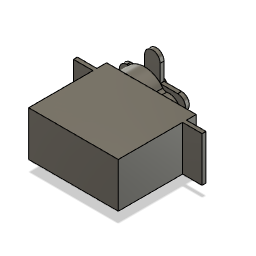
Pan_Tilt_Assembly (Autodesk Fusion 360 archive; units mm, degrees)
design "Servo9gr"
Autodesk Fusion 360 part; units mm, degrees
sketch "Skizze1" plane through (0, 0, 0) normal (0, 0, 1) x (1, 0, 0)
  line L0 (11.5, 5.75) -> (-11.5, 5.75)
  line L1 (-11.5, 5.75) -> (-11.5, -5.75)
  line L2 (-11.5, -5.75) -> (11.5, -5.75)
  line L3 (11.5, -5.75) -> (11.5, 5.75)
  line L4 (11.5, 5.75) -> (-11.5, -5.75) construction
  line L5 (-11.5, 5.75) -> (11.5, -5.75) construction
  dimension "d1" = 11.5
  dimension "d2" = 23
  constraint horizontal L0
  constraint perpendicular L0 L1
  constraint parallel L0 L2
  constraint parallel L1 L3
  constraint coincident L4 origin
  constraint coincident L5 origin
  measures "d1" distance of L0.start L2.end
  measures "d2" distance of L0.start L0.end
extrude "Extrusion1" add sketch "Skizze1" along normal mid plane 20
sketch "Skizze2" plane through (0, 5.75, 0) normal (0, 1, 0) x (-1, 0, 0)
  line L0 (11.5, -10) -> (11.5, 10)
  line L1 (11.5, 10) -> (-11.5, 10)
  line L2 (-11.5, 10) -> (-11.5, -10)
  line L3 (-11.5, -10) -> (11.5, -10)
  line L4 (16.5, -7.5) -> (-16.5, -7.5)
  line L5 (-16.5, -7.5) -> (-16.5, -6.5)
  line L6 (-16.5, -6.5) -> (16.5, -6.5)
  line L7 (16.5, -6.5) -> (16.5, -7.5)
  dimension "d5" = 2.5
  dimension "d6" = 1
  dimension "d7" = 5
  dimension "d8" = 5
  constraint horizontal L4
  constraint vertical L5
  constraint horizontal L6
  constraint vertical L7
  measures "d5" distance of L3 L4
  measures "d6" distance of L4.end L5.end
  measures "d7" distance of L2 L5
  measures "d8" distance of L0 L7
extrude "Extrusion2" add sketch "Skizze2" against normal blind 11.5 contours L0 L4 L6 L7 | L2 L4 L5 L6
sketch "Skizze3" plane through (0, 0, -10) normal (0, 0, -1) x (-1, 0, 0)
  line L0 (-11.5, 5.75) -> (-11.5, -5.75)
  line L1 (-11.5, -5.75) -> (11.5, -5.75)
  line L2 (11.5, -5.75) -> (11.5, 5.75)
  line L3 (11.5, 5.75) -> (-11.5, 5.75)
  circle A0 centre (5.75, 0) radius 5.75
  circle A1 centre (-0.5, 0) radius 3
  dimension "d11" = 11.5
  dimension "d13" = 6
  dimension "d14" = 12
  constraint tangent L3 A0
  constraint tangent L1 A0
  constraint tangent L2 A0
  measures "d11" diameter of A0
  measures "d13" diameter of A1
  measures "d14" distance of L2 A1.centre
extrude "Extrusion3" add sketch "Skizze3" along normal blind 4 contours A0 A1 | A0 A1 | A0 A1
fillet "Abrundung1" radius 1 2 edges at (-0.7, 2.7495, -12) (-0.7, -2.7495, -12)
sketch "Skizze4" plane through (0, 0, -14) normal (0, 0, -1) x (-1, 0, 0)
  arc A0 (1.0733, -3.3453) -> (1.0733, 3.3453) centre (5.75, 0) ccw
  arc A1 (0.07, 2.9454) -> (1.0733, 3.3453) centre (0.26, 3.9271) ccw
  arc A2 (0.07, 2.9454) -> (0.07, -2.9454) centre (-0.5, 0) ccw
  arc A3 (1.0733, -3.3453) -> (0.07, -2.9454) centre (0.26, -3.9271) ccw
  circle A4 centre (5.75, 0) radius 2.5
  dimension "d19" = 5
  constraint concentric A0 A4
  measures "d19" diameter of A4
extrude "Extrusion4" add sketch "Skizze4" along normal blind 2 contours A4
sketch "Skizze5" plane through (0, 0, -16) normal (0, 0, -1) x (-1, 0, 0)
  circle A0 centre (5.75, 0) radius 2.5
  line L0 (7.75, 8.5) -> (3.75, 8.5)
  line L1 (3.75, -8.5) -> (7.75, -8.5)
  line L2 (7.75, 8.5) -> (3.75, -8.5) construction
  line L3 (3.75, 8.5) -> (7.75, -8.5) construction
  line L4 (-2.75, 2) -> (-2.75, -2)
  line L5 (14.25, -2) -> (14.25, 2)
  line L6 (14.25, 2) -> (-2.75, -2) construction
  line L7 (-2.75, 2) -> (14.25, -2) construction
  line L8 (3.75, 2) -> (-2.75, 2)
  line L9 (3.75, 8.5) -> (3.75, 2)
  line L10 (3.75, 0.4706) -> (3.75, -0.4706)
  line L11 (3.75, -2) -> (3.75, -8.5)
  line L12 (-2.75, -2) -> (3.75, -2)
  line L13 (7.75, -2) -> (14.25, -2)
  line L14 (7.75, -8.5) -> (7.75, -2)
  line L15 (7.75, -0.4706) -> (7.75, 0.4706)
  line L16 (7.75, 2) -> (7.75, 8.5)
  line L17 (14.25, 2) -> (7.75, 2)
  line L18 (6.2206, 2) -> (5.2794, 2)
  point P0 (5.75, 0)
  point P1 (5.75, 0)
  dimension "d22" = 4
  dimension "d23" = 17
  constraint horizontal L0
  constraint perpendicular L0 L9
  constraint parallel L0 L1
  constraint parallel L9 L14
  constraint coincident L2 P1
  constraint coincident L3 P1
  constraint coincident P0 A0.centre
  constraint horizontal L17
  constraint perpendicular L4 L17
  constraint parallel L12 L17
  constraint parallel L4 L5
  constraint coincident L6 P1
  constraint coincident L7 P1
  constraint coincident P1 P0
  constraint equal L0 L5
  constraint coincident L3 L18.end
  constraint collinear L8 L17
  constraint collinear L9 L10
  constraint coincident L7 L10.start
  constraint coincident L6 L10.end
  constraint collinear L10 L11
  constraint collinear L12 L13
  constraint collinear L14 L15
  constraint coincident L7 L15.start
  constraint coincident L6 L15.end
  constraint collinear L15 L16
  constraint collinear L17 L18
  constraint coincident L2 L18.start
  measures "d22" distance of L0.start L0.end
  measures "d23" distance of L0.start L1.end
extrude "Extrusion5" add sketch "Skizze5" along normal blind 1 contours A0 | L0 L1 L4 L5 L8 L9 L11 L12 L13 L14 L16 L17
fillet "Abrundung2" radius 2 8 edges at (2.75, -2, -16.5) (-3.75, -8.5, -16.5) (-7.75, -8.5, -16.5) (-14.25, -2, -16.5) (-14.25, 2, -16.5) (-7.75, 8.5, -16.5) (-3.75, 8.5, -16.5) (2.75, 2, -16.5)
sketch "Skizze6" plane through (0, 0, -17) normal (0, 0, -1) x (-1, 0, 0)
  arc A0 (-0.75, 2) -> (-0.75, -2) centre (-0.75, 0) ccw
  line L0 (-0.75, -2) -> (3.75, -2)
  line L1 (3.75, -2) -> (3.75, -6.5)
  arc A1 (3.75, -6.5) -> (7.75, -6.5) centre (5.75, -6.5) ccw
  line L2 (7.75, -6.5) -> (7.75, -2)
  line L3 (7.75, -2) -> (12.25, -2)
  arc A2 (12.25, -2) -> (12.25, 2) centre (12.25, 0) ccw
  line L4 (12.25, 2) -> (7.75, 2)
  line L5 (7.75, 2) -> (7.75, 6.5)
  arc A3 (7.75, 6.5) -> (3.75, 6.5) centre (5.75, 6.5) ccw
  line L6 (3.75, 6.5) -> (3.75, 2)
  line L7 (3.75, 2) -> (-0.75, 2)
  line L8 (5.75, 6.5) -> (5.75, -6.5) construction
  line L9 (12.25, 0) -> (-0.75, 0) construction
  circle A4 centre (5.75, 0) radius 2
  dimension "d28" = 4
  constraint coincident A3.centre L8.start
  constraint coincident A1.centre L8.end
  constraint coincident A2.centre L9.start
  constraint coincident A0.centre L9.end
  constraint coincident L8 A4.centre
  constraint coincident L9 A4.centre
  measures "d28" diameter of A4
extrude "Extrusion6" add sketch "Skizze6" along normal blind 1 contours A4
sketch "Skizze7" plane through (-11.5, 0, 0) normal (-1, 0, 0) x (0, 0, 1)
  line L0 (-6.5, 5.75) -> (-6.5, -5.75)
  line L1 (-6.5, -5.75) -> (10, -5.75)
  line L2 (10, -5.75) -> (10, 5.75)
  line L3 (10, 5.75) -> (-6.5, 5.75)
  ellipse E0 centre (6, 0) end of major axis (6, 2.5) minor radius 1.5
  line L4 (6, -2.5) -> (6, 2.5)
  line L5 (7.5, 0) -> (4.5, 0)
  dimension "d31" = 5
  dimension "d32" = 3
  dimension "d33" = 4
  constraint coincident E0 L4.start
  constraint coincident E0 L4.end
  constraint coincident E0 L5.start
  constraint coincident E0 L5.end
  constraint vertical L4
  constraint horizontal origin E0.centre
  measures "d31" distance of E0
  measures "d33" distance of L2 L4
extrude "Extrusion7" add sketch "Skizze7" along normal blind 2 contours E0 L4 L5 | E0 L4 L5 | E0 L4 L5 | E0 L4 L5
equation "d8 = d7"

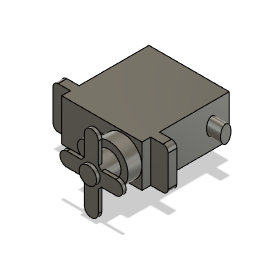
design "Servo180"
Autodesk Fusion 360 part; units mm, degrees
sketch "Skizze1" plane through (0, 0, 0) normal (0, 0, 1) x (1, 0, 0)
  line L0 (11.5, 6) -> (-11.5, 6)
  line L1 (-11.5, 6) -> (-11.5, -6)
  line L2 (-11.5, -6) -> (11.5, -6)
  line L3 (11.5, -6) -> (11.5, 6)
  line L4 (11.5, 6) -> (-11.5, -6) construction
  line L5 (-11.5, 6) -> (11.5, -6) construction
  dimension "d1" = 23
  dimension "d2" = 12
  constraint horizontal L0
  constraint perpendicular L0 L1
  constraint parallel L0 L2
  constraint parallel L1 L3
  constraint coincident L4 origin
  constraint coincident L5 origin
  measures "d1" distance of L1.end L2.end
  measures "d2" distance of L0.end L1.end
extrude "Extrusion1" add sketch "Skizze1" along normal mid plane 25
sketch "Skizze2" plane through (0, -6, 0) normal (0, -1, 0) x (1, 0, 0)
  line L0 (11.5, -12.5) -> (11.5, 12.5)
  line L1 (11.5, 12.5) -> (-11.5, 12.5)
  line L2 (-11.5, 12.5) -> (-11.5, -12.5)
  line L3 (-11.5, -12.5) -> (11.5, -12.5)
  line L4 (-16.5, 10) -> (16.5, 10)
  line L5 (16.5, 10) -> (16.5, 7.5)
  line L6 (16.5, 7.5) -> (-16.5, 7.5)
  line L7 (-16.5, 7.5) -> (-16.5, 10)
  dimension "d5" = 2.5
  dimension "d6" = 2.5
  dimension "d7" = 5
  dimension "d8" = 5
  constraint horizontal L4
  constraint vertical L5
  constraint horizontal L6
  constraint vertical L7
  measures "d5" distance of L1 L4
  measures "d6" distance of L4 L6
  measures "d7" distance of L2 L7
  measures "d8" distance of L0 L5
extrude "Extrusion2" add sketch "Skizze2" against normal blind 12 contours L0 L4 L5 L6 | L2 L4 L6 L7
fillet "Abrundung1" radius 1.5 4 edges at (16.5, -6, 8.75) (16.5, 6, 8.75) (-16.5, -6, 8.75) (-16.5, 6, 8.75)
sketch "Skizze3" plane through (0, 0, 12.5) normal (0, 0, 1) x (1, 0, 0)
  line L0 (11.5, -6) -> (11.5, 6)
  line L1 (11.5, 6) -> (-11.5, 6)
  line L2 (-11.5, 6) -> (-11.5, -6)
  line L3 (-11.5, -6) -> (11.5, -6)
  circle A0 centre (6, 0) radius 5.5
  circle A1 centre (-0.5, 0) radius 2.5
  dimension "d13" = 11
  dimension "d15" = 5
  dimension "d16" = 12
  constraint horizontal origin A0.centre
  constraint tangent L0 A0
  constraint horizontal origin A1.centre
  measures "d13" diameter of A0
  measures "d15" diameter of A1
  measures "d16" distance of L0 A1.centre
extrude "Extrusion3" add sketch "Skizze3" along normal blind 4 contours A0 A1 | A0 A1 | A0 A1
fillet "Abrundung2" radius 1 2 edges at (0.9038, -2.0686, 14.5) (0.9038, 2.0686, 14.5)
sketch "Skizze4" plane through (11.5, 0, 0) normal (1, 0, 0) x (0, 0, -1)
  line L0 (-7.5, 6) -> (-7.5, -6)
  line L1 (-7.5, -6) -> (12.5, -6)
  line L2 (12.5, -6) -> (12.5, 6)
  line L3 (12.5, 6) -> (-7.5, 6)
  ellipse E0 centre (7.5, 0) end of major axis (7.5, 2.5) minor radius 1.5
  line L4 (7.5, -2.5) -> (7.5, 2.5)
  line L5 (9, 0) -> (6, 0)
  dimension "d21" = 5
  dimension "d22" = 3
  dimension "d23" = 5
  constraint coincident E0 L4.start
  constraint coincident E0 L4.end
  constraint coincident E0 L5.start
  constraint coincident E0 L5.end
  constraint parallel L0 L4
  constraint horizontal origin E0.centre
  measures "d21" distance of E0
  measures "d23" distance of L2 L4
extrude "Extrusion4" add sketch "Skizze4" along normal blind 4 contours E0 L4 L5 | E0 L4 L5 | E0 L4 L5 | E0 L4 L5
sketch "Skizze5" plane through (0, 0, 16.5) normal (0, 0, 1) x (1, 0, 0)
  arc A0 (1.2973, -2.8522) -> (1.2973, 2.8522) centre (6, 0) ccw
  arc A1 (0.1731, 2.4077) -> (1.2973, 2.8522) centre (0.4423, 3.3708) ccw
  arc A2 (0.1731, 2.4077) -> (0.1731, -2.4077) centre (-0.5, 0) ccw
  arc A3 (1.2973, -2.8522) -> (0.1731, -2.4077) centre (0.4423, -3.3708) ccw
  circle A4 centre (6, 0) radius 3.5
  dimension "d26" = 7
  constraint concentric A0 A4
  measures "d26" diameter of A4
extrude "Extrusion5" add sketch "Skizze5" along normal blind 4 contours A4
sketch "Skizze6" plane through (0, 0, 20.5) normal (0, 0, 1) x (1, 0, 0)
  circle A0 centre (6, 0) radius 3.5
  line L0 (8, 11) -> (4, 11)
  line L1 (4, -11) -> (8, -11)
  line L2 (8, 11) -> (4, -11) construction
  line L3 (4, 11) -> (8, -11) construction
  line L4 (-3, -2) -> (-3, 2)
  line L5 (15, 2) -> (15, -2)
  line L6 (15, -2) -> (-3, 2) construction
  line L7 (-3, -2) -> (15, 2) construction
  line L8 (-3, 2) -> (3.1277, 2)
  line L9 (5.6364, 2) -> (6.3636, 2)
  line L10 (8.8723, 2) -> (15, 2)
  line L11 (4, 11) -> (4, 2.8723)
  line L12 (8, 2.8723) -> (8, 11)
  line L13 (8, -11) -> (8, -2)
  line L14 (8, -0.4444) -> (8, 0.4444)
  line L15 (15, -2) -> (8.8723, -2)
  line L16 (6.3636, -2) -> (5.6364, -2)
  line L17 (3.1277, -2) -> (-3, -2)
  line L18 (4, 0.4444) -> (4, -0.4444)
  line L19 (4, -2.8723) -> (4, -11)
  point P0 (6, 0)
  point P1 (6, 0)
  dimension "d29" = 4
  dimension "d30" = 4
  dimension "d31" = 18
  dimension "d32" = 22
  constraint horizontal L0
  constraint perpendicular L0 L11
  constraint parallel L0 L1
  constraint parallel L11 L13
  constraint coincident L2 P1
  constraint coincident L3 P1
  constraint coincident P0 A0.centre
  constraint horizontal L15
  constraint perpendicular L4 L15
  constraint parallel L8 L15
  constraint parallel L4 L5
  constraint coincident L6 P1
  constraint coincident L7 P1
  constraint coincident L3 L9.start
  constraint collinear L8 L9
  constraint coincident L2 L9.end
  constraint collinear L9 L10
  constraint coincident A0 L8.end
  constraint coincident A0 L11.end
  constraint coincident L6 L18.start
  constraint collinear L11 L18
  constraint coincident A0 L10.start
  constraint coincident L7 L14.end
  constraint coincident A0 L12.start
  constraint collinear L12 L13
  constraint coincident L13.end L15
  constraint coincident L6 L14.start
  constraint collinear L13 L14
  constraint coincident A0 L15.end
  constraint collinear L15 L16
  constraint coincident L2 L16.end
  constraint collinear L16 L17
  constraint coincident A0 L17.start
  constraint coincident L7 L18.end
  constraint coincident A0 L19.start
  constraint collinear L18 L19
  constraint coincident L3 L16.start
  measures "d29" distance of L0.start L0.end
  measures "d30" distance of L5.end L5.start
  measures "d31" distance of L4 L5
  measures "d32" distance of L0 L1
extrude "Extrusion6" add sketch "Skizze6" along normal blind 1
fillet "Abrundung3" radius 2 8 edges at (-3, -2, 21) (4, -11, 21) (8, -11, 21) (15, -2, 21) (15, 2, 21) (8, 11, 21) (4, 11, 21) (-3, 2, 21)
sketch "Skizze7" plane through (0, 0, 21.5) normal (0, 0, 1) x (1, 0, 0)
  arc A0 (-1, 2) -> (-1, -2) centre (-1, 0) ccw
  line L0 (-1, -2) -> (3.1277, -2)
  arc A1 (3.1277, -2) -> (4, -2.8723) centre (6, 0) ccw
  line L1 (4, -2.8723) -> (4, -9)
  arc A2 (4, -9) -> (8, -9) centre (6, -9) ccw
  line L2 (8, -9) -> (8, -2.8723)
  arc A3 (8, -2.8723) -> (8.8723, -2) centre (6, 0) ccw
  line L3 (8.8723, -2) -> (13, -2)
  arc A4 (13, -2) -> (13, 2) centre (13, 0) ccw
  line L4 (13, 2) -> (8.8723, 2)
  arc A5 (8.8723, 2) -> (8, 2.8723) centre (6, 0) ccw
  line L5 (8, 2.8723) -> (8, 9)
  arc A6 (8, 9) -> (4, 9) centre (6, 9) ccw
  line L6 (4, 9) -> (4, 2.8723)
  arc A7 (4, 2.8723) -> (3.1277, 2) centre (6, 0) ccw
  line L7 (3.1277, 2) -> (-1, 2)
  circle A8 centre (6, 0) radius 2.5
  dimension "d37" = 5
  constraint concentric A1 A8
  measures "d37" diameter of A8
extrude "Extrusion7" add sketch "Skizze7" along normal blind 1 contours A8
equation "d8 = d7"
equation "d30 = d29"
